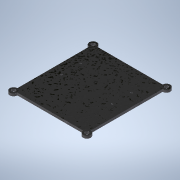
# Autodesk Inventor part: base
Saved by Autodesk Inventor 2021 (Build 250183000, 183)
## iProperties
Created: 2021-03-04
Part Number: base
Material: Steel, Mild, Welded
Document SubType Name: Modeling
Designer: Usuario
Density: 7.85 g/cm^3
Appearance: Weld - Steel Mild
Author: Usuario
Autodesk Inventor part; units mm, degrees
ref_plane "YZ Plane" through (0, 0, 0) normal (1, 0, 0) x (0, 1, 0)
ref_plane "XZ Plane" through (0, 0, 0) normal (0, 1, 0) x (-1, 0, 0)
ref_plane "XY Plane" through (0, 0, 0) normal (0, 0, 1) x (1, 0, 0)
sketch "Sketch1" plane through (0, 0, 0) normal (0, 1, 0) x (-1, 0, 0)
  line L0 (0, 0) -> (65, 0)
  line L1 (65, 0) -> (65, -70)
  line L2 (65, -70) -> (0, -70)
  line L3 (0, -70) -> (0, 0)
  dimension "d0" = 65
  dimension "d1" = 70
  constraints: 8 end point, 2 parallel, 1 horizontal, 1 perpendicular
  measures "d0" distance of L1.end L2.end
  measures "d1" distance of L0.end L1.end
extrude "Extrusion1" add sketch "Sketch1" along normal blind 2
sketch "Sketch2" plane through (0, 2, 0) normal (0, 1, 0) x (1, 0, 0)
  line L0 (0, 70) -> (-65, 70) projected
  line L1 (-32.5, 69) -> (-10.5, 69)
  line L2 (-32.5, 69) -> (-54.5, 69)
  line L3 (-10.5, 69) -> (-10.5, 55)
  line L4 (-10.5, 55) -> (-54.5, 55)
  line L5 (-54.5, 55) -> (-54.5, 69)
  line L6 (-65, 0) -> (0, 0) projected
  line L7 (-32.4987, 3) -> (-20.9987, 3)
  line L8 (-32.4987, 3) -> (-43.9987, 3)
  line L9 (-11.55, 31.8) -> (-55, 31.8)
  line L10 (-11.55, 31.8) -> (-11.55, 50)
  line L11 (-55, 31.8) -> (-55, 50)
  line L12 (-55, 50) -> (-11.55, 50)
  line L13 (-20.9987, 3) -> (-20.9987, 19)
  line L14 (-20.9987, 19) -> (-43.9987, 19)
  line L15 (-43.9987, 19) -> (-43.9987, 3)
  line L16 (-20.9987, 19) -> (-20.9987, 16.39)
  line L17 (-20.9987, 19) -> (-20.9987, 16.08)
  line L18 (-55, 50) -> (-53.73, 50)
  circle A0 centre (-53.73, 48.73) radius 0.635
  circle A1 centre (-53.73, 33.07) radius 0.635
  circle A2 centre (-12.82, 48.73) radius 0.635
  circle A3 centre (-12.82, 33.07) radius 0.635
  point P0 (-2, 70)
  point P1 (-63, 70)
  point P2 (-63, 0)
  point P3 (-2, 0)
  dimension "d20" = 18.2
  dimension "d27" = 23
  dimension "d54" = 1.27
  dimension "d56" = 1.27
  dimension "d58" = 1.27
  dimension "d60" = 43.45
  dimension "d63" = 1.27
  dimension "d64" = 1.27
  constraints: 34 end point, 5 perpendicular, 4 centre point, 3 horizontal, 3 point on line, 3 vertical
  measures "d20" distance of L9.end L11.end
  measures "d27" distance of L13.end L14.end
  measures "d54" distance of L11.end L18.end
  measures "d56" diameter of A0
  measures "d58" diameter of A1
  measures "d60" distance of L9.start L9.end
  measures "d63" diameter of A2
  measures "d64" diameter of A3
extrude "Extrusion2" cut sketch "Sketch2" against normal blind 2 contours A0 | A1 | A2 | A3
sketch "Sketch4" plane through (0, 2, 0) normal (0, 1, 0) x (1, 0, 0)
  arc A0 (-63, 70) -> (-65, 68) centre (-63, 68) ccw projected
  line L0 (-63, 68) -> (-61.5, 68) construction
  circle A1 centre (-61.9393, 66.9393) radius 1.5
  arc A2 (0, 68) -> (-2, 70) centre (-2, 68) ccw projected
  arc A3 (-65, 2) -> (-63, 0) centre (-63, 2) ccw projected
  arc A4 (-2, 0) -> (0, 2) centre (-2, 2) ccw projected
  line L1 (-2, 68) -> (-0.5, 68) construction
  circle A5 centre (-3.0607, 66.9393) radius 1.5
  line L2 (-63, 2) -> (-61.5, 2) construction
  circle A6 centre (-61.9393, 3.0607) radius 1.5
  arc A7 (-2, 0) -> (0, 2) centre (-2, 2) ccw projected
  line L3 (-2, 2) -> (-0.5, 2) construction
  circle A8 centre (-3.0607, 3.0607) radius 1.5
  point P0 (0, 0)
  dimension "d69" = 3
  dimension "d72" = 3
  dimension "d75" = 3
  dimension "d78" = 3
  constraints: 8 end point, 4 centre point, 4 horizontal
  measures "d69" diameter of A1
  measures "d72" diameter of A5
  measures "d75" diameter of A6
  measures "d78" diameter of A8
extrude "Extrusion3" cut sketch "Sketch4" against normal blind 2
sketch "Sketch5" plane through (0, 2, 0) normal (0, 1, 0) x (1, 0, 0)
  circle A0 centre (-3.0607, 3.0607) radius 1.5 projected
  circle A1 centre (-3.0607, 66.9393) radius 1.5 projected
  circle A2 centre (-61.9393, 3.0607) radius 1.5 projected
  circle A3 centre (-61.9393, 66.9393) radius 1.5 projected
  circle A4 centre (-12.82, 48.73) radius 0.635 projected
  circle A5 centre (-53.73, 33.07) radius 0.635 projected
  circle A6 centre (-12.82, 33.07) radius 0.635 projected
  circle A7 centre (-53.73, 48.73) radius 0.635 projected
  line L0 (-65, 70) -> (-65, 0) projected
  line L1 (-65, 0) -> (0, 0) projected
  line L2 (0, 0) -> (0, 70) projected
  line L3 (0, 70) -> (-65, 70) projected
  circle A8 centre (-61.9393, 3.0607) radius 1.5 projected
  circle A9 centre (-3.0607, 66.9393) radius 1.5 projected
  line L4 (-61.9393, 3.0607) -> (-3.0607, 3.0607)
  line L5 (-3.0607, 3.0607) -> (-3.0607, 66.9393)
  line L6 (-3.0607, 66.9393) -> (-61.9393, 66.9393)
  line L7 (-61.9393, 66.9393) -> (-61.9393, 3.0607)
  circle A10 centre (-61.9393, 3.0607) radius 3.0607
  line L8 (-65, 0) -> (0, 0) projected
  circle A11 centre (-61.9393, 66.9393) radius 1.5 projected
  circle A12 centre (-61.9393, 66.9393) radius 3.0607
  line L9 (0, 70) -> (-65, 70) projected
  circle A13 centre (-3.0607, 66.9393) radius 1.5 projected
  circle A14 centre (-3.0607, 66.9393) radius 3.0607
  circle A15 centre (-3.0607, 3.0607) radius 1.5 projected
  circle A16 centre (-3.0607, 3.0607) radius 3.0607
  line L10 (0, 0) -> (0, 70) projected
  line L11 (0, 3.0607) -> (0, 0)
  line L12 (0, 0) -> (-3.0607, 0)
  line L13 (0, 66.9393) -> (0, 70)
  line L14 (0, 70) -> (-3.0607, 70)
  line L15 (-65, 70) -> (-65, 0) projected
  line L16 (-61.9393, 70) -> (-65, 70)
  line L17 (-65, 70) -> (-65, 66.9393)
  line L18 (-65, 3.0607) -> (-65, 0)
  line L19 (-65, 0) -> (-61.9393, 0)
  point P0 (-3.0607, 0)
  constraints: 24 end point, 8 point on circle, 8 point on line, 5 tangent, 4 centre point, 4 coincident, 3 collinear, 2 horizontal, 2 parallel, 1 perpendicular
extrude "Extrusion4" cut sketch "Sketch5" against normal blind 2 contours L2 L1 A16 | A14 L3 L2 | L1 L0 A10 | A12 L0 L3
sketch "Sketch6" plane through (0, 2, 0) normal (0, 1, 0) x (1, 0, 0)
  arc A0 (0, 66.9393) -> (-3.0607, 70) centre (-3.0607, 66.9393) ccw projected
  line L0 (-3.0607, 70) -> (-61.9393, 70) projected
  arc A1 (-61.9393, 70) -> (-65, 66.9393) centre (-61.9393, 66.9393) ccw projected
  line L1 (-65, 66.9393) -> (-65, 3.0607) projected
  arc A2 (-65, 3.0607) -> (-61.9393, 0) centre (-61.9393, 3.0607) ccw projected
  line L2 (-61.9393, 0) -> (-3.0607, 0) projected
  arc A3 (-3.0607, 0) -> (0, 3.0607) centre (-3.0607, 3.0607) ccw projected
  line L3 (0, 3.0607) -> (0, 66.9393) projected
  circle A4 centre (-3.0607, 3.0607) radius 1.5 projected
  circle A5 centre (-3.0607, 66.9393) radius 1.5 projected
  circle A6 centre (-61.9393, 3.0607) radius 1.5 projected
  circle A7 centre (-61.9393, 66.9393) radius 1.5 projected
  circle A8 centre (-12.82, 48.73) radius 0.635 projected
  circle A9 centre (-53.73, 33.07) radius 0.635 projected
  circle A10 centre (-12.82, 33.07) radius 0.635 projected
  circle A11 centre (-53.73, 48.73) radius 0.635 projected
  circle A12 centre (-3.0607, 66.9393) radius 3.0607
  circle A13 centre (-3.0607, 3.0607) radius 1.5 projected
  circle A14 centre (-3.0607, 3.0607) radius 3.0607
  circle A15 centre (-61.9393, 3.0607) radius 1.5 projected
  circle A16 centre (-61.9393, 3.0607) radius 3.0607
  circle A17 centre (-61.9393, 66.9393) radius 1.5 projected
  circle A18 centre (-61.9393, 66.9393) radius 3.0607
  line L4 (-58.8787, 3.0607) -> (-6.1213, 3.0607)
  line L5 (-3.0607, 6.1213) -> (-3.0607, 63.8787)
  line L6 (-6.1213, 66.9393) -> (-58.8787, 66.9393)
  line L7 (-61.9393, 63.8787) -> (-61.9393, 6.1213)
  arc A19 (-65, 3.0607) -> (-61.9393, 0) centre (-61.9393, 3.0607) ccw projected
  line L8 (-61.9393, 0) -> (-3.0607, 0)
  line L9 (-61.9393, 0) -> (-3.0607, 0) projected
  line L10 (-65, 3.0607) -> (-65, 66.9393)
  line L11 (-3.0607, 70) -> (-61.9393, 70) projected
  line L12 (-61.9393, 70) -> (-3.0607, 70)
  arc A20 (0, 66.9393) -> (-3.0607, 70) centre (-3.0607, 66.9393) ccw projected
  line L13 (0, 3.0607) -> (0, 66.9393) projected
  line L14 (0, 3.0607) -> (0, 66.9393)
  point P0 (0, 0)
  point P1 (-65, 3.0607)
  point P2 (-3.0607, 0)
  constraints: 16 end point, 10 point on circle, 4 centre point, 4 coincident, 4 perpendicular, 2 collinear, 1 concentric, 1 vertical
extrude "Extrusion5" cut sketch "Sketch6" against normal blind 2 contours L3 A14 L5 A12 | A12 L6 A18 L0 | L2 A16 L4 A14 | A18 L7 A16 L1
body "Solid1"
